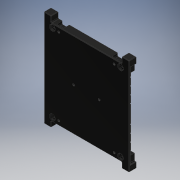
# Autodesk Inventor part: +Y
Saved by Autodesk Inventor 2018 (Build 220112000, 112)
## iProperties
Created: 2018-07-04
Part Number: +Y
Material: Aluminum 6061
Document SubType Name: Modeling
Designer: Bradley
Density: 2.7 g/cm^3
Appearance: Anodized - Dark Gray
Mass: 115.419 g
Surface Area: 282.423 cm^2
Volume: 42.7479 cm^3
Author: Bradley
Autodesk Inventor part; units mm, degrees
ref_plane "YZ Plane" through (0, 0, 0) normal (1, 0, 0) x (0, 1, 0)
ref_plane "XZ Plane" through (0, 0, 0) normal (0, 1, 0) x (-1, 0, 0)
ref_plane "XY Plane" through (0, 0, 0) normal (0, 0, 1) x (1, 0, 0)
sketch "Sketch1" plane through (0, 0, 0) normal (0, 1, 0) x (-1, 0, 0)
  line L0 (50, 57) -> (50, -56.5)
  line L1 (50, -56.5) -> (41.5, -56.5)
  line L2 (41.5, -56.5) -> (41.5, -50)
  line L3 (41.5, -50) -> (-41.5, -50)
  line L4 (-41.5, -50) -> (-41.5, -56.5)
  line L5 (-41.5, -56.5) -> (-50, -56.5)
  line L6 (-50, -56.5) -> (-50, 57)
  line L7 (-50, 57) -> (-41.5, 57)
  line L8 (-41.5, 57) -> (-41.5, 50)
  line L9 (-41.5, 50) -> (41.5, 50)
  line L10 (41.5, 50) -> (41.5, 57)
  line L11 (50, 57) -> (41.5, 57)
  point P0 (0, 0)
  point P1 (0, 50)
  dimension "d0" = 100
  dimension "d1" = 8.5
  dimension "d2" = 113.5
  dimension "d3" = 7
  dimension "d4" = 6.5
  dimension "d5" = 56.5
  constraints: 24 end point, 8 perpendicular, 7 point on line, 1 collinear, 1 midpoint, 1 vertical, 1 vertical alignment
  measures "d0" distance between parallel lines of L6 L0
  measures "d1" distance of L0.start L10.end
  measures "d2" distance of L0.start L0.end
  measures "d3" distance of L9.end L10.end
  measures "d4" distance of L1.end L2.end
  measures "d5" distance from line of point (0, 0) L1
extrude "Extrusion1" add sketch "Sketch1" along normal mid plane 8.5
sketch "Sketch2" plane through (50, -4.25, -56.5) normal (1, 0, 0) x (0, 0, -1)
  line L0 (0, 8.5) -> (0, 0) projected
  line L1 (-113.5, 8.5) -> (0, 8.5) projected
  line L2 (-113.5, 8.5) -> (-113.5, 0) projected
  line L3 (0, 0) -> (-113.5, 0) projected
  line L4 (0, 8.5) -> (-113.5, 8.5) projected
  line L5 (-98.5, 8.5) -> (-98.5, 4)
  line L6 (-98.5, 4) -> (-14.5, 4)
  line L7 (-14.5, 4) -> (-14.5, 8.5)
  line L8 (-46.55, 4) -> (-45.45, 4)
  line L9 (-45.45, 4) -> (-45.45, 2)
  line L10 (-45.45, 2) -> (-46.55, 2)
  line L11 (-46.55, 2) -> (-46.55, 4)
  line L12 (-113.5, 0) -> (0, 0) construction
  line L13 (-56.5, 0) -> (-56.5, 8.5) construction
  line L14 (-37.55, 2) -> (-37.55, 4)
  line L15 (-37.55, 4) -> (-36.45, 4)
  line L16 (-36.45, 2) -> (-37.55, 2)
  line L17 (-36.45, 4) -> (-36.45, 2)
  line L18 (-28.55, 2) -> (-28.55, 4)
  line L19 (-28.55, 4) -> (-27.45, 4)
  line L20 (-27.45, 2) -> (-28.55, 2)
  line L21 (-27.45, 4) -> (-27.45, 2)
  line L22 (-19.55, 2) -> (-19.55, 4)
  line L23 (-19.55, 4) -> (-18.45, 4)
  line L24 (-18.45, 2) -> (-19.55, 2)
  line L25 (-18.45, 4) -> (-18.45, 2)
  line L26 (-66.45, 4) -> (-67.55, 4)
  line L27 (-67.55, 4) -> (-67.55, 2)
  line L28 (-67.55, 2) -> (-66.45, 2)
  line L29 (-66.45, 2) -> (-66.45, 4)
  line L30 (-75.45, 2) -> (-75.45, 4)
  line L31 (-75.45, 4) -> (-76.55, 4)
  line L32 (-76.55, 2) -> (-75.45, 2)
  line L33 (-76.55, 4) -> (-76.55, 2)
  line L34 (-84.45, 2) -> (-84.45, 4)
  line L35 (-84.45, 4) -> (-85.55, 4)
  line L36 (-85.55, 2) -> (-84.45, 2)
  line L37 (-85.55, 4) -> (-85.55, 2)
  line L38 (-93.45, 2) -> (-93.45, 4)
  line L39 (-93.45, 4) -> (-94.55, 4)
  line L40 (-94.55, 2) -> (-93.45, 2)
  line L41 (-94.55, 4) -> (-94.55, 2)
  line L42 (-106.5, 8.5) -> (-106.5, 0) projected
  line L43 (-6.5, 8.5) -> (-6.5, 0) projected
  point P0 (-56.5, 4.25)
  point P1 (-46, 2)
  point P2 (-37, 2)
  point P3 (-28, 2)
  point P4 (-19, 2)
  point P5 (-67, 2)
  point P6 (-76, 2)
  point P7 (-85, 2)
  point P8 (-94, 2)
  dimension "d26" = 0.5
  dimension "d8" = 4
  dimension "d11" = 1.1
  dimension "d12" = 2
  dimension "d15" = 9
  dimension "d20" = 21
  dimension "d23" = 8
  dimension "d24" = 8
  dimension "d80" = 4.5
  constraints: 72 end point, 20 symmetric about line, 5 point on line, 4 perpendicular, 2 horizontal, 2 midpoint, 2 parallel, 1 vertical, 27 other
  measures "d8" distance between parallel lines of L6 L3
  measures "d11" distance of L9.end L10.end
  measures "d12" distance between parallel lines of L10 L3
  measures "d15" distance of L8.start L14.end
  measures "d20" distance of point (-46, 2) point (-67, 2)
  measures "d23" distance between parallel lines of L43 L7
  measures "d24" distance between parallel lines of L5 L42
  measures "d80" distance from line of point (-94, 2) L5
extrude "Extrusion2" cut sketch "Sketch2" against normal through all contours L7 L6 L5 L1 | L25 L24 L22 L6 | L6 L38 L40 L41 | L21 L20 L18 L6 | L6 L34 L36 L37 | L17 L16 L14 L6 | L6 L30 L32 L33 | L9 L10 L11 L6 | L6 L29 L28 L27
fillet "Fillet1" radius 1 6 edges at (41.5, 0, 50) (-41.5, 0, 50) (-41.5, 0, -50) (41.5, 0, -50) (50, -4.25, 0.25) (-50, -4.25, 0.25)
chamfer "Chamfer1" distance 0.5 angle 45 30 edges at (-45.25, -4.25, 57) (-49.7071, -3.9571, 57) (-50, 0.5, 57) (-45.75, 4.25, 57) (-41.5, 0, 57) (0, -4.25, 50) (-41.2071, -4.25, 50.2929) (-41.5, -4.25, 54) (41.2071, -4.25, 50.2929) (41.5, -4.25, 54) (41.5, 0, 57) (45.25, -4.25, 57) (49.7071, -3.9571, 57) (50, 0.5, 57) (45.75, 4.25, 57) (45.25, -4.25, -56.5) (49.7071, -3.9571, -56.5) (50, 0.5, -56.5) (45.75, 4.25, -56.5) (41.5, 0, -56.5) (41.5, -4.25, -53.75) (41.2071, -4.25, -50.2929) (0, -4.25, -50) (-41.2071, -4.25, -50.2929) (-41.5, -4.25, -53.75) (-45.75, 4.25, -56.5) (-50, 0.5, -56.5) (-49.7071, -3.9571, -56.5) (-45.25, -4.25, -56.5) (-41.5, 0, -56.5)
sketch "Sketch3" plane through (0, -4.25, 0) normal (0, -1, 0) x (1, 0, 0)
  line L0 (32.5, -45) -> (-32.5, -45) construction
  line L1 (-32.5, -45) -> (-32.5, 45) construction
  line L2 (-32.5, 45) -> (32.5, 45) construction
  line L3 (32.5, 45) -> (32.5, -45) construction
  line L4 (32.5, -45) -> (-32.5, 45) construction
  line L5 (-32.5, -45) -> (32.5, 45) construction
  line L6 (-15, 0) -> (15, 0) construction
  point P0 (0, 0)
  point P1 (0, 0)
  dimension "d29" = 65
  dimension "d30" = 90
  dimension "d31" = 30
  constraints: 14 end point, 6 coincident, 4 midpoint, 2 horizontal, 2 parallel, 1 perpendicular
  measures "d29" distance of L1.end L2.end
  measures "d30" distance of L0.end L1.end
  measures "d31" distance of L6.start L6.end
hole "Hole1" at (-32.5, -4.25, 45) at (32.5, -4.25, 45) at (32.5, -4.25, -45) at (-32.5, -4.25, -45) at (-15, -4.25, 0) at (15, -4.25, 0) direction (0, 1, 0) diameter 2.621 end through all thread size "M3x0.35" class "6H" standard "ANSI Metric M Profile"
sketch "Sketch4" plane through (0, 4.25, 0) normal (0, 1, 0) x (1, 0, 0)
  circle A0 centre (-32.5, -45) radius 1.3105 projected
  line L0 (50, -42) -> (-50, -42) projected
  line L1 (-50, -42) -> (-50, -56.5) projected
  line L2 (-41.5, -56.5) -> (-50, -56.5) projected
  line L3 (50, -56.5) -> (41.5, -56.5) projected
  line L4 (50, -56.5) -> (50, -42) projected
  circle A1 centre (32.5, -45) radius 1.3105 projected
  line L5 (-36.55, -50) -> (-28.45, -50)
  line L6 (-28.45, -50) -> (-28.45, -46.95)
  line L7 (-28.45, -46.95) -> (-36.55, -46.95)
  line L8 (-36.55, -46.95) -> (-36.55, -50)
  line L9 (36.55, -50) -> (28.45, -50)
  line L10 (28.45, -50) -> (28.45, -46.95)
  line L11 (28.45, -46.95) -> (36.55, -46.95)
  line L12 (36.55, -46.95) -> (36.55, -50)
  line L13 (0, -50) -> (0, -44) construction
  line L14 (15, -47) -> (-15, -47) construction
  line L15 (15, -45.45) -> (-15, -45.45)
  line L16 (-15, -48.55) -> (15, -48.55)
  arc A2 (15, -48.55) -> (15, -45.45) centre (15, -47) ccw
  arc A3 (-15, -45.45) -> (-15, -48.55) centre (-15, -47) ccw
  line L17 (-41.5, -56.5) -> (-41.5, -51) projected
  arc A4 (-40.5, -50) -> (-41.5, -51) centre (-40.5, -51) ccw projected
  line L18 (-40.5, -50) -> (40.5, -50) projected
  arc A5 (41.5, -51) -> (40.5, -50) centre (40.5, -51) ccw projected
  line L19 (41.5, -51) -> (41.5, -56.5) projected
  point P0 (0, 0)
  point P1 (-32.5, -46.95)
  point P2 (0, -47)
  dimension "d39" = 3.05
  dimension "d40" = 8.1
  dimension "d42" = 30
  dimension "d43" = 3.1
  constraints: 26 end point, 5 midpoint, 5 parallel, 4 point on circle, 4 tangent, 3 perpendicular, 3 point on line, 2 centre point, 2 horizontal, 1 vertical alignment, 2 other
  measures "d39" distance of L7.end L5.start
  measures "d40" distance of L6.end L7.end
  measures "d42" distance of L14.start L14.end
  measures "d43" distance between parallel lines of L15 L16
extrude "Extrusion3" cut sketch "Sketch4" against normal blind 3.1 contours A2 L16 A3 L15
extrude "Extrusion4" cut sketch "Sketch4" against normal blind 6.6 contours L9 L10 L11 L12 | L8 L7 L6 L5
sketch "Sketch5" plane through (0, -4.25, 0) normal (0, -1, 0) x (1, 0, 0)
  circle A0 centre (-15, 0) radius 1.3105 projected
  circle A1 centre (32.5, -45) radius 1.3105 projected
  circle A2 centre (-32.5, 45) radius 1.3105 projected
  circle A3 centre (32.5, 45) radius 1.3105 projected
  circle A4 centre (-32.5, -45) radius 1.3105 projected
  circle A5 centre (15, 0) radius 1.3105 projected
  line L0 (49, -56) -> (42, -56) projected
  line L1 (49, 56.5) -> (49, -56) projected
  line L2 (42, 56.5) -> (49, 56.5) projected
  line L3 (42, 51) -> (42, 56.5) projected
  arc A6 (40.5, 49.5) -> (42, 51) centre (40.5, 51) ccw projected
  line L4 (-40.5, 49.5) -> (40.5, 49.5) projected
  arc A7 (-42, 51) -> (-40.5, 49.5) centre (-40.5, 51) ccw projected
  line L5 (-42, 56.5) -> (-42, 51) projected
  line L6 (-49, 56.5) -> (-42, 56.5) projected
  line L7 (-49, -56) -> (-49, 56.5) projected
  line L8 (-42, -56) -> (-49, -56) projected
  line L9 (-42, -51) -> (-42, -56) projected
  arc A8 (-40.5, -49.5) -> (-42, -51) centre (-40.5, -51) ccw projected
  line L10 (40.5, -49.5) -> (-40.5, -49.5) projected
  arc A9 (42, -51) -> (40.5, -49.5) centre (40.5, -51) ccw projected
  line L11 (42, -56) -> (42, -51) projected
  line L12 (28.45, 46.95) -> (36.55, 46.95) projected
  line L13 (28.45, 50) -> (28.45, 46.95) projected
  line L14 (36.55, 50) -> (28.45, 50) projected
  line L15 (36.55, 46.95) -> (36.55, 50) projected
  line L16 (50, 42) -> (-50, 42) projected
  circle A10 centre (40, 45.5) radius 3 construction
  line L17 (40, 45.5) -> (-40, 45.5) construction
  point P0 (0, 0)
  point P1 (33.347, 44)
  point P2 (0, 45.5)
  dimension "d52" = 6
  dimension "d53" = 4.5
  dimension "d54" = 80
  constraints: 2 coincident, 2 end point, 1 centre point, 1 horizontal, 1 midpoint, 1 vertical alignment, 2 other
  measures "d52" diameter of A10
  measures "d53" distance from line of L17.start L14
  measures "d54" distance of L17.start L17.end
hole "Hole2" at (-40, -4.25, 45.5) at (40, -4.25, 45.5) direction (0, 1, 0) diameter 3.2 end through all counterbore diameter 6 counterbore depth 2.1 clearance for "Socket Head Cap Screw" size "M3" standard "Ansi Metric M Profile"
mirror "Mirror2" about plane through (0, 0, 0) normal (0, 0, 1) of "Hole2", "Extrusion3"
fillet "Fillet3" radius 1 4 edges at (36.55, 0.95, 46.95) (28.45, 0.95, 46.95) (-36.55, 0.95, 46.95) (-28.45, 0.95, 46.95)
chamfer "Chamfer3" distance 0.5 angle 45 22 edges at (32.5, 4.25, 46.95) (36.2571, 4.25, 47.2429) (36.55, 4.25, 48.975) (28.7429, 4.25, 47.2429) (28.45, 4.25, 48.975) (-16.55, 4.25, 47) (0, 4.25, 45.45) (16.55, 4.25, 47) (0, 4.25, 48.55) (-28.7429, 4.25, 47.2429) (-32.5, 4.25, 46.95) (-36.2571, 4.25, 47.2429) (-36.55, 4.25, 48.975) (-28.45, 4.25, 48.975) (-16.55, 4.25, -47) (0, 4.25, -48.55) (16.55, 4.25, -47) (0, 4.25, -45.45) (40, -4.25, 48.5) (-40, -4.25, 48.5) (40, -4.25, -48.5) (-40, -4.25, -48.5)
sketch "Sketch6" plane through (50, -0.25, -42) normal (1, 0, 0) x (0, 0, -1)
  line L0 (14, 4.5) -> (14, -3) projected
  line L1 (0, 4.5) -> (14, 4.5) projected
  line L2 (0, 4.5) -> (0, 0) projected
  line L3 (0, 0) -> (-3.95, 0) projected
  line L4 (-3.95, 0) -> (-3.95, -2) projected
  line L5 (-3.95, -2) -> (-5.05, -2) projected
  line L6 (-5.05, -2) -> (-5.05, 0) projected
  line L7 (-5.05, 0) -> (-12.95, 0) projected
  line L8 (-12.95, 0) -> (-12.95, -2) projected
  line L9 (-12.95, -2) -> (-14.05, -2) projected
  line L10 (-14.05, -2) -> (-14.05, 0) projected
  line L11 (-14.05, 0) -> (-21.95, 0) projected
  line L12 (-21.95, 0) -> (-21.95, -2) projected
  line L13 (-21.95, -2) -> (-23.05, -2) projected
  line L14 (-23.05, -2) -> (-23.05, 0) projected
  line L15 (-23.05, 0) -> (-30.95, 0) projected
  line L16 (-30.95, 0) -> (-30.95, -2) projected
  line L17 (-30.95, -2) -> (-32.05, -2) projected
  line L18 (-32.05, -2) -> (-32.05, 0) projected
  line L19 (-32.05, 0) -> (-51.95, 0) projected
  line L20 (-51.95, 0) -> (-51.95, -2) projected
  line L21 (-51.95, -2) -> (-53.05, -2) projected
  line L22 (-53.05, -2) -> (-53.05, 0) projected
  line L23 (-53.05, 0) -> (-60.95, 0) projected
  line L24 (-60.95, 0) -> (-60.95, -2) projected
  line L25 (-60.95, -2) -> (-62.05, -2) projected
  line L26 (-62.05, -2) -> (-62.05, 0) projected
  line L27 (-62.05, 0) -> (-69.95, 0) projected
  line L28 (-69.95, 0) -> (-69.95, -2) projected
  line L29 (-69.95, -2) -> (-71.05, -2) projected
  line L30 (-71.05, -2) -> (-71.05, 0) projected
  line L31 (-71.05, 0) -> (-78.95, 0) projected
  line L32 (-78.95, 0) -> (-78.95, -2) projected
  line L33 (-78.95, -2) -> (-80.05, -2) projected
  line L34 (-80.05, -2) -> (-80.05, 0) projected
  line L35 (-80.05, 0) -> (-84, 0) projected
  line L36 (-84, 0) -> (-84, 4.5) projected
  line L37 (-98.5, 4.5) -> (-84, 4.5) projected
  line L38 (-98.5, -3) -> (-98.5, 4.5) projected
  line L39 (14, -3) -> (-98.5, -3) projected
  line L40 (-92.05, 4.5) -> (-92.05, -2.55)
  line L41 (-92.05, -2.55) -> (8.05, -2.55)
  line L42 (8.05, -2.55) -> (8.05, 4.5)
  line L43 (0, 4.5) -> (14, 4.5) projected
  line L44 (-98.5, 46) -> (14, 46) construction
  line L45 (-98.5, -4) -> (14, -4) projected
  point P0 (-42, 0.25)
  point P1 (-42, -2.55)
  dimension "d66" = 50
  dimension "d67" = 97.1
  dimension "d69" = 100.1
  constraints: 8 end point, 3 vertical alignment, 2 perpendicular, 2 point on line, 1 horizontal, 1 midpoint
  measures "d66" distance between parallel lines of L44 L45
  measures "d67" diameter of L41 L44
  measures "d69" distance of L40.end L41.end
extrude "Extrusion5" cut sketch "Sketch6" against normal blind 2 contours L42 L41 L40 L37 L36 L35 L34 L33 L32 L31 L30 L29 L28 L27 L26 L25 L24 L23 L22 L21 L20 L19 L18 L17 L16 L15 L14 L13 L12 L11 L10 L9 L8 L7 L6 L5 L4 L3 L2 L1
mirror "Mirror3" about plane through (0, 0, 0) normal (1, 0, 0) of "Extrusion5"
fillet "Fillet4" radius 1 4 edges at (-48, 0.725, 50.05) (-48, 0.725, -50.05) (48, 0.725, 50.05) (48, 0.725, -50.05)
sketch "Sketch7" plane through (49.5, 3.75, -56.5) normal (0, 0, -1) x (-1, 0, 0)
  line L0 (7.5, 0) -> (7.5, -7.5) projected
  line L1 (0, 0) -> (7.5, 0) projected
  line L2 (0, -7) -> (0, 0) projected
  arc A0 (0, -7) -> (0.5, -7.5) centre (0.5, -7) ccw projected
  line L3 (7.5, -7.5) -> (0.5, -7.5) projected
  point P0 (49.5, -3.75)
  point P1 (4, -3.5)
  point P2 (4, -7.5)
  point P3 (0, -3.5)
  constraints: 2 midpoint, 1 horizontal alignment, 1 vertical alignment
hole "Hole3" at (45.5, 0.25, -56.5) direction (0, 0, 1) diameter 3.404 depth 12.5 tip angle 118 thread size "8-36 UNF" class "2B" standard "ANSI Unified Screw Threads"
equation "\"d23\" = d24"
body "Solid1"
